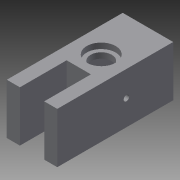
# Autodesk Inventor part: Cubeta Final sin huecos
Saved by Autodesk Inventor 2014 (Build 180170000, 170)
## iProperties
Created: 2015-03-26
Part Number: Cubeta Final sin huecos
Material: Genérico
Document SubType Name: Modeling
Designer: HP
Density: 1 g/cm^3
Appearance: Valor por defecto
Author: HP
Autodesk Inventor part; units mm, degrees
ref_plane "YZ Plane" through (0, 0, 0) normal (1, 0, 0) x (0, 1, 0)
ref_plane "XZ Plane" through (0, 0, 0) normal (0, 1, 0) x (-1, 0, 0)
ref_plane "XY Plane" through (0, 0, 0) normal (0, 0, 1) x (1, 0, 0)
sketch "Boceto1" plane through (0, 0, 0) normal (0, 1, 0) x (-1, 0, 0)
  line L0 (-19.9533, 14.4643) -> (7.0467, 14.4643)
  line L1 (7.0467, 14.4643) -> (7.0467, -12.5357)
  line L2 (7.0467, -12.5357) -> (-19.9533, -12.5357)
  line L3 (-19.9533, -12.5357) -> (-19.9533, 14.4643)
  point P0 (0, 0)
  dimension "d0" = 27
  dimension "d1" = 27
  constraints: 8 end point, 2 parallel, 1 horizontal, 1 perpendicular
  measures "d0" distance of L0.end L1.end
  measures "d1" distance of L1.end L2.end
extrude "Extrusión1" add sketch "Boceto1" along normal blind 62
sketch "Boceto2" plane through (0, 62, 0) normal (0, 1, 0) x (1, 0, 0)
  line L0 (-7.0467, -14.4643) -> (19.9533, -14.4643) projected
  line L1 (19.9533, -14.4643) -> (19.9533, 12.5357) projected
  line L2 (19.9533, 12.5357) -> (-7.0467, 12.5357) projected
  line L3 (-7.0467, 12.5357) -> (-7.0467, -14.4643) projected
  line L4 (-1.0467, 6.5357) -> (13.9533, 6.5357)
  line L5 (13.9533, 6.5357) -> (13.9533, -8.4643)
  line L6 (13.9533, -8.4643) -> (-1.0467, -8.4643)
  line L7 (-1.0467, -8.4643) -> (-1.0467, 6.5357)
  point P0 (0, 0)
  dimension "d4" = 6
  dimension "d5" = 6
  dimension "d6" = 6
  dimension "d7" = 6
  constraints: 8 end point, 2 parallel, 1 horizontal, 1 perpendicular
  measures "d4" distance between parallel lines of L1 L5
  measures "d5" distance between parallel lines of L2 L4
  measures "d6" distance between parallel lines of L3 L7
  measures "d7" distance between parallel lines of L6 L0
extrude "Extrusión2" cut sketch "Boceto2" against normal blind 31 contours L4 L5 L6 L7
sketch "Boceto3" plane through (19.9533, 0, -12.5357) normal (0, 0, -1) x (-1, 0, 0)
  line L0 (27, 0) -> (0, 0) projected
  line L1 (27, 0) -> (27, 62) projected
  line L2 (0, 0) -> (0, 62) projected
  line L3 (20, 25) -> (7, 25)
  line L4 (7, 25) -> (7, 0)
  line L5 (7, 0) -> (20, 0)
  line L6 (20, 0) -> (20, 25)
  line L7 (0, 62) -> (27, 62) projected
  circle A0 centre (13.5, 39) radius 2.55
  point P0 (19.9533, 0)
  dimension "d10" = 7
  dimension "d11" = 7
  dimension "d12" = 25
  dimension "d16" = 5.1
  dimension "d17" = 13.5
  dimension "d18" = 23
  constraints: 8 end point, 2 parallel, 1 centre point, 1 horizontal, 1 perpendicular, 1 point on line
  measures "d10" distance between parallel lines of L2 L4
  measures "d11" distance between parallel lines of L6 L1
  measures "d12" distance of L5.end L3.start
  measures "d16" diameter of A0
  measures "d17" distance from line of L2 A0.centre
  measures "d18" distance from line of L7 A0.centre
extrude "Extrusión3" cut sketch "Boceto3" against normal blind 30 contours L0 L4 L3 L6
sketch "Boceto4" plane through (19.9533, 62, -12.5357) normal (0, 0, -1) x (-1, 0, 0)
  line L0 (0, -62) -> (0, 0) projected
  circle A0 centre (13.5, -25) radius 1.55
  line L1 (21, -31) -> (6, -31) projected
  point P0 (19.9533, -62)
  dimension "d19" = 3.1
  dimension "d20" = 13.5
  dimension "d34" = 6
  constraints: 1 centre point
  measures "d19" diameter of A0
  measures "d20" distance from line of A0.centre L0
  measures "d34" distance from line of L1 A0.centre
extrude "Extrusión4" cut sketch "Boceto4" against normal blind 7
sketch "Boceto5" plane through (-7.0467, 62, 14.4643) normal (0, 0, 1) x (1, 0, 0)
  line L0 (27, -62) -> (27, 0) projected
  circle A0 centre (13.5, -25) radius 7.75
  line L1 (21, -31) -> (6, -31) projected
  point P0 (7.0467, -62)
  dimension "d24" = 15.5
  dimension "d25" = 13.5
  dimension "d33" = 6
  constraints: 1 centre point
  measures "d24" diameter of A0
  measures "d25" distance from line of L0 A0.centre
  measures "d33" distance from line of L1 A0.centre
extrude "Extrusión5" cut sketch "Boceto5" against normal blind 3
sketch "Boceto6" plane through (6.4533, 37, 11.4643) normal (0, 0, 1) x (1, 0, 0)
  circle A0 centre (0, 0) radius 7.75 projected
  circle A1 centre (0, 0) radius 5.65
  point P0 (-6.4533, -37)
  dimension "d29" = 11.3
  constraints: 1 centre point, 1 coincident
  measures "d29" diameter of A1
extrude "Extrusión6" cut sketch "Boceto6" against normal blind 3 contours A1
sketch "Boceto8" plane through (-7.0467, 0, -12.5357) normal (-1, 0, 0) x (0, 0, 1)
  line L0 (27, 0) -> (27, 62) projected
  circle A0 centre (13.5, 37) radius 1.5
  line L1 (0, 25) -> (27, 25) projected
  line L2 (0, 25) -> (27, 25) projected
  point P0 (12.5357, 0)
  dimension "d42" = 13.5
  dimension "d43" = 3
  dimension "d47" = 12
  constraints: 1 centre point
  measures "d42" distance from line of L0 A0.centre
  measures "d43" diameter of A0
  measures "d47" distance from line of L2 A0.centre
extrude "Extrusión8" cut sketch "Boceto8" against normal through all
sketch "Boceto10" plane through (0, 31, 0) normal (0, 1, 0) x (1, 0, 0)
  line L0 (-1.0467, 6.5357) -> (13.9533, 6.5357) projected
  line L1 (13.9533, 6.5357) -> (13.9533, -8.4643) projected
  circle A0 centre (6.4533, -0.9643) radius 1.5
  point P0 (0, 0)
  dimension "d62" = 3
  dimension "d63" = 7.5
  dimension "d64" = 7.5
  constraints: 1 centre point
  measures "d62" diameter of A0
  measures "d63" distance from line of L0 A0.centre
  measures "d64" distance from line of L1 A0.centre
extrude "Extrusión10" cut sketch "Boceto10" against normal through all
